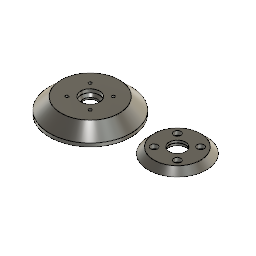
Oberteil (Autodesk Fusion 360 design; units mm, degrees)
Autodesk Fusion 360 part; units mm, degrees
sketch "Skizze1" plane through (0, 0, 0) normal (0, 0, 1) x (1, 0, 0)
  circle A0 centre (0, 0) radius 35
  dimension "d1" = 70
  measures "d1" diameter of A0
extrude "Extrusion1" add sketch "Skizze1" along normal blind 3 makes body 1
sketch "Skizze2" plane through (0, 0, 0) normal (0, 0, 1) x (1, 0, 0)
  line L0 (18.9028, -18.9028) -> (28.3542, -9.4514)
  line L1 (28.3542, -9.4514) -> (28.3542, 9.4514)
  line L2 (28.3542, 9.4514) -> (18.9028, 18.9028)
  line L3 (-18.9028, 18.9028) -> (-28.3542, 9.4744)
  line L4 (-28.3542, 9.4744) -> (-28.3542, -9.4514)
  line L5 (-28.3542, -9.4514) -> (-18.9258, -18.9028)
  line L6 (-20, 20) -> (-30, 9.8026)
  line L7 (-30, 9.8026) -> (-30, -10)
  line L8 (-30, -10) -> (-19.9463, -20)
  line L9 (-19.9463, -20) -> (20, -20)
  line L10 (20, -20) -> (30, -10)
  line L11 (30, -10) -> (30, 10)
  line L12 (30, 10) -> (20, 20)
  line L13 (20, 20) -> (-20, 20)
  line L14 (-19.3102, -18.5175) -> (19.2881, -18.5175)
  line L15 (19.2881, 18.5175) -> (-19.2891, 18.5175)
extrude "Extrusion2" add sketch "Skizze2" against normal blind 1.5 separate body makes body 2
sketch "Skizze3" plane through (0, 0, 0) normal (0, 0, -1) x (1, 0, 0)
  circle A0 centre (0, 0) radius 35
  line L0 (-25, 7.9838) -> (-18, 15)
  line L1 (-18, 15) -> (18.2597, 15)
  line L2 (18.2597, 15) -> (25, 8)
  line L3 (25, 8) -> (25, -8)
  line L4 (25, -8) -> (18.2597, -15)
  line L5 (18.2597, -15) -> (-18, -15)
  line L6 (-18, -15) -> (-25, -8)
  line L7 (-25, 7.9838) -> (-25, -8)
ref_plane "Arbeitsebene1" through (0, 0, 13) normal (0, 0, 1) x (1, 0, 0)
sketch "Skizze4" plane through (0, 0, 13) normal (0, 0, 1) x (1, 0, 0)
  circle A0 centre (0, 0) radius 25
  dimension "d13" = 50
  measures "d13" diameter of A0
loft "Erhebung1" add profiles "Skizze4" section 1 face at (8.8451, -11.8425, 3) section 2 on bodies 1 bodies 1
extrude "Extrusion3" cut sketch "Skizze3" against normal blind 6.5 contours L0 L1 L2 L3 L4 L5 L6 L7 bodies 1
chamfer "Fase1" distance 3.03 angle 65 8 edges at (0.1298, -15, 0) (21.6298, -11.5, 0) (25, 0, 0) (21.6298, 11.5, 0) (0.1298, 15, 0) (-21.5, 11.5, 0) (-25, 0.0081, 0) (-21.5, -11.4919, 0) measured on face at (0.9584, -21.634, 0) measured on face at (0.9584, -21.634, 0) measured on face at (0.9584, -21.634, 0) measured on face at (0.9584, -21.634, 0) measured on face at (0.9584, -21.634, 0) measured on face at (0.9584, -21.634, 0) measured on face at (0.9584, -21.634, 0) measured on face at (0.9584, -21.634, 0) on bodies 1
sketch "Skizze5" plane through (0, 0, 6.5) normal (0, 0, -1) x (1, 0, 0)
  line L0 (-18, 15) -> (-25, 7.9838)
  line L1 (-25, 7.9838) -> (-25, -8)
  line L2 (-25, -8) -> (-18, -15)
  line L3 (-18, -15) -> (18.2597, -15)
  line L4 (18.2597, -15) -> (25, -8)
  line L5 (25, -8) -> (25, 8)
  line L6 (25, 8) -> (18.2597, 15)
  line L7 (18.2597, 15) -> (-18, 15)
  circle A0 centre (0, 0) radius 6
  dimension "d18" = 12
  measures "d18" diameter of A0
extrude "Extrusion4" cut sketch "Skizze5" against normal blind 10 contours A0 bodies 1
sketch "Skizze6" plane through (0, 0, 13) normal (0, 0, 1) x (-1, 0, 0)
  circle A0 centre (0, 0) radius 6
  circle A1 centre (0, 0) radius 25
  circle A2 centre (0, 0) radius 8.1
  dimension "d21" = 16.2
  measures "d21" diameter of A2
extrude "Extrusion5" cut sketch "Skizze6" against normal blind 3 contours A2 bodies 1
sketch "Skizze7" plane through (0, 0, 13) normal (0, 0, 1) x (-1, 0, 0)
  circle A0 centre (0, 0) radius 8.1
  circle A1 centre (0, 0) radius 25
  circle A2 centre (10, -10) radius 1.25
  circle A3 centre (-10, -10) radius 1.25
  circle A4 centre (10, 10) radius 1.25
  circle A5 centre (-10, 10) radius 1.25
  dimension "d26" = 2.5
  dimension "d27" = 2.5
  dimension "d28" = 2.5
  dimension "d29" = 2.5
  measures "d26" diameter of A2
  measures "d27" diameter of A3
  measures "d28" diameter of A4
  measures "d29" diameter of A5
extrude "Extrusion6" cut sketch "Skizze7" against normal blind 5 contours A2 | A3 | A4 | A5 bodies 1
sketch "Skizze8" plane through (0, 0, 0) normal (0, 0, -1) x (1, 0, 0)
  circle A0 centre (0, 0) radius 35
  line L0 (-28.03, -9.2551) -> (-28.03, 9.2369)
  line L1 (-28.03, 9.2369) -> (-19.2571, 18.03)
  line L2 (-19.2571, 18.03) -> (19.5484, 18.03)
  line L3 (19.5484, 18.03) -> (28.03, 9.2217)
  line L4 (28.03, 9.2217) -> (28.03, -9.2217)
  line L5 (28.03, -9.2217) -> (19.5484, -18.03)
  line L6 (19.5484, -18.03) -> (-19.2551, -18.03)
  line L7 (-19.2551, -18.03) -> (-28.03, -9.2551)
  circle A1 centre (-15, 25) radius 1.25
  circle A2 centre (15, 25) radius 1.25
  circle A3 centre (-15, -25) radius 1.25
  circle A4 centre (15, -25) radius 1.25
  dimension "d32" = 30
  dimension "d33" = 50
  dimension "d34" = 2.5
  dimension "d35" = 2.5
  dimension "d36" = 2.5
  dimension "d37" = 2.5
  measures "d34" diameter of A1
  measures "d35" diameter of A2
  measures "d36" diameter of A3
  measures "d37" diameter of A4
extrude "Extrusion7" cut sketch "Skizze8" against normal blind 6 contours A1 | A2 | A3 | A4 bodies 1
sketch "Skizze9" plane through (0, 0, 0) normal (0, 0, 1) x (1, 0, 0)
  circle A0 centre (75, 0) radius 25
  dimension "d42" = 50
  measures "d42" diameter of A0
ref_plane "Arbeitsebene3" through (75, 0, 5) normal (0, 0, 1) x (1, 0, 0)
sketch "Skizze13" plane through (75, 0, 5) normal (0, 0, 1) x (1, 0, 0)
  circle A0 centre (0, 0) radius 20
  dimension "d46" = 40
  measures "d46" diameter of A0
loft "Erhebung2" add profiles "Skizze13", "Skizze9" section 1 section 2 separate body makes body 3
sketch "Skizze14" plane through (0, 0, 5) normal (0, 0, 1) x (-1, 0, 0)
  circle A0 centre (-75, 0) radius 20
  circle A1 centre (-65, -10) radius 1.5
  circle A2 centre (-85, -10) radius 1.5
  circle A3 centre (-65, 10) radius 1.5
  circle A4 centre (-85, 10) radius 1.5
  dimension "d47" = 20
  dimension "d48" = 20
  dimension "d49" = 3
  dimension "d50" = 3
  dimension "d51" = 3
  dimension "d52" = 3
  measures "d49" diameter of A1
  measures "d50" diameter of A2
  measures "d51" diameter of A3
  measures "d52" diameter of A4
extrude "Extrusion8" cut sketch "Skizze14" against normal blind 8 contours A1 | A2 | A3 | A4 bodies 3
sketch "Skizze15" plane through (0, 0, 5) normal (0, 0, 1) x (-1, 0, 0)
  circle A0 centre (-85, -10) radius 1.5
  circle A1 centre (-85, 10) radius 1.5
  circle A2 centre (-65, -10) radius 1.5
  circle A3 centre (-65, 10) radius 1.5
  circle A4 centre (-75, 0) radius 20
  circle A5 centre (-65, -10) radius 3
  circle A6 centre (-85, -10) radius 3
  circle A7 centre (-65, 10) radius 3
  circle A8 centre (-85, 10) radius 3
  dimension "d55" = 6
  dimension "d56" = 6
  dimension "d57" = 6
  dimension "d58" = 6
  measures "d55" diameter of A5
  measures "d56" diameter of A6
  measures "d57" diameter of A7
  measures "d58" diameter of A8
extrude "Extrusion9" cut sketch "Skizze15" against normal blind 3.5 contours A5 | A6 | A7 | A8 bodies 3
sketch "Skizze16" plane through (0, 0, 5) normal (0, 0, 1) x (-1, 0, 0)
  circle A0 centre (-85, -10) radius 3
  circle A1 centre (-85, 10) radius 3
  circle A2 centre (-65, -10) radius 3
  circle A3 centre (-65, 10) radius 3
  circle A4 centre (-75, 0) radius 20
  circle A5 centre (-75, 0) radius 7
  dimension "d61" = 14
  measures "d61" diameter of A5
extrude "Extrusion10" cut sketch "Skizze16" against normal blind 8 contours A5 bodies 3
sketch "Skizze17" plane through (0, 0, 0) normal (0, 0, -1) x (1, 0, 0)
  circle A0 centre (75, 0) radius 7
  circle A1 centre (85, -10) radius 1.5
  circle A2 centre (85, 10) radius 1.5
  circle A3 centre (65, -10) radius 1.5
  circle A4 centre (65, 10) radius 1.5
  circle A5 centre (75, 0) radius 25
  circle A6 centre (75, 0) radius 8.1
  dimension "d64" = 16.2
  measures "d64" diameter of A6
extrude "Extrusion11" cut sketch "Skizze17" against normal blind 2 contours A6 bodies 3
move_body "Verschieben1" bodies 3 to x (1, 0, 0) y (0, 1, 0) z (0, 0, 1) at (0, 0, 8)
chamfer "Fase3" distance 2 angle 45 1 edges at (-5.594, -2.1697, 10) on bodies 1
chamfer "Fase4" distance 1 angle 45 1 edges at (81.5263, -2.5313, 10) on bodies 3
